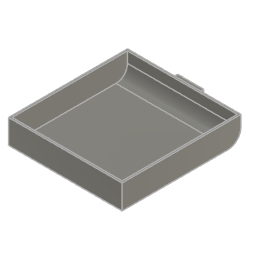
Drawer (Autodesk Fusion 360 design; units mm, degrees)
Autodesk Fusion 360 part; units mm, degrees
sketch "Sketch1" plane through (0, 9.525, 0) normal (0, 1, 0) x (-1, 0, 0)
  line L0 (40.0034, -41.91) -> (40.0034, -46.99)
  line L1 (40.0034, -46.99) -> (150.4934, -46.99)
  line L2 (150.4934, -46.99) -> (150.4934, -41.91)
  line L3 (150.4934, -41.91) -> (175.8934, -41.91)
  line L4 (175.8934, -41.91) -> (175.8934, -6.985)
  line L5 (175.8934, -6.985) -> (14.6034, -6.985)
  line L6 (14.6034, -6.985) -> (14.6034, -41.91)
  line L7 (14.6034, -41.91) -> (40.0034, -41.91)
  line L8 (40.3534, -46.64) -> (150.1434, -46.64)
  line L9 (150.1434, -46.64) -> (150.1434, -41.56)
  line L10 (150.1434, -41.56) -> (175.5434, -41.56)
  line L11 (175.5434, -41.56) -> (175.5434, -7.335)
  line L12 (175.5434, -7.335) -> (14.9534, -7.335)
  line L13 (14.9534, -7.335) -> (14.9534, -41.56)
  line L14 (14.9534, -41.56) -> (40.3534, -41.56)
  line L15 (40.3534, -41.56) -> (40.3534, -46.64)
  line L16 (40.3534, -41.56) -> (150.1434, -41.56)
  dimension "d105" = -0.35
extrude "Extrude1" add sketch "Sketch1" along normal up to surface (168.275 mm away) contours L10 L11 L12 L13 L14 L16
fillet "Fillet2" chord length 26.67 tangency weight 1.05 1 edges at (-95.2484, 177.8, -41.56)
shell "Shell2" thickness 2.54 removed faces 1 at (-122.0134, 65.6167, -7.335)
sketch "Sketch2" plane through (0, 177.8, 0) normal (0, 1, 0) x (-1, 0, 0)
  line L0 (175.5434, -22.7015) -> (14.9534, -22.7015)
  line L1 (175.5434, -22.7015) -> (175.5434, -7.335)
  line L2 (175.5434, -7.335) -> (14.9534, -7.335)
  line L3 (14.9534, -7.335) -> (14.9534, -22.7015)
  line L4 (14.9534, -15.0182) -> (175.5434, -15.0182) construction
  line L5 (95.2484, -7.335) -> (95.2484, -22.7015) construction
  line L6 (76.8334, -12.1607) -> (82.5484, -12.1607)
  line L7 (82.5484, -12.1607) -> (82.5484, -17.8757)
  line L8 (82.5484, -17.8757) -> (76.8334, -17.8757)
  line L9 (76.8334, -17.8757) -> (76.8334, -12.1607)
  line L10 (76.8334, -12.1607) -> (82.5484, -17.8757) construction
  line L11 (82.5484, -12.1607) -> (76.8334, -17.8757) construction
  line L12 (107.9484, -12.1607) -> (107.9484, -17.8757)
  line L13 (113.6634, -12.1607) -> (107.9484, -12.1607)
  line L14 (113.6634, -17.8757) -> (113.6634, -12.1607)
  line L15 (107.9484, -17.8757) -> (113.6634, -17.8757)
  point P0 (79.6909, -15.0182)
  dimension "d122" = 5.715
  dimension "d123" = 5.715
  dimension "d124" = 12.7
  constraint midpoint L3 L4.start
  constraint midpoint L1 L4.end
  constraint midpoint L2 L5.start
  constraint midpoint L0 L5.end
  constraint horizontal L6
  constraint perpendicular L6 L7
  constraint parallel L6 L8
  constraint parallel L7 L9
  constraint coincident L10 P0
  constraint coincident L11 P0
  constraint coincident L4 P0
  constraint symmetric L5 L6.start L13.start
  constraint symmetric L5 L6.end L12.start
  constraint symmetric L5 L7.end L12.end
  constraint symmetric L5 L8.end L14.start
  measures "d122" distance of L7.end L8.end
  measures "d123" distance of L6.end L7.end
  measures "d124" distance of L5 L7
ref_plane "WorkPlane1" through (-95.2484, 93.6625, -14.955) normal (0, 0, 1) x (1, 0, 0)
sketch "Sketch3" plane through (0, 0, -14.955) normal (0, 0, 1) x (1, 0, 0)
  line L0 (-113.6634, 177.8) -> (-107.9484, 177.8)
  line L1 (-79.6909, 177.8) -> (-79.6909, 184.1413)
  line L2 (-79.6909, 184.1413) -> (-110.8059, 184.1413)
  line L3 (-110.8059, 184.1413) -> (-110.8059, 177.8)
  point P0 (-79.6909, 177.8)
  point P1 (-110.8059, 177.8)
  constraint midpoint L0 P1
  constraint coincident P0 L1.start
  constraint vertical L1
  constraint perpendicular L1 L2
  constraint coincident P1 L3.end
  constraint perpendicular L0 L3
sweep "Sweep1" add profiles "Sketch2" path "Sketch3" along L1 L2 L3 section 1 contours L6 L7 L8 L9
